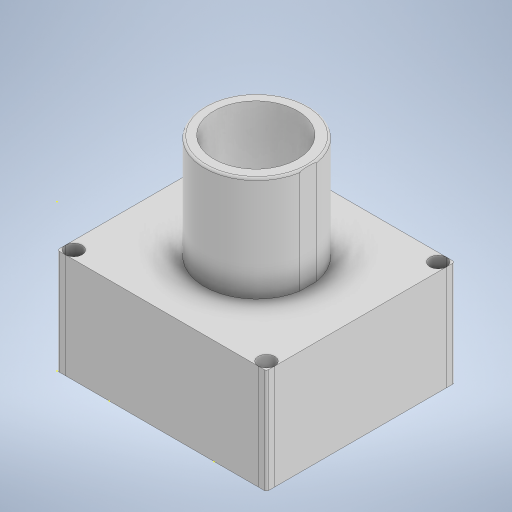
# Autodesk Inventor part: TAREA1_AR
Saved by Autodesk Inventor 2024 (Build 280153000, 153)
## iProperties
Created: 2024-02-15
Part Number: TAREA1_AR
Material: Generic
Document SubType Name: Modeling
Designer: Andreita
Density: 1 g/cm^3
Appearance: Default
Author: Andreita
Autodesk Inventor part; units mm, degrees
ref_plane "YZ Plane" through (0, 0, 0) normal (1, 0, 0) x (0, 1, 0)
ref_plane "XZ Plane" through (0, 0, 0) normal (0, 1, 0) x (-1, 0, 0)
ref_plane "XY Plane" through (0, 0, 0) normal (0, 0, 1) x (1, 0, 0)
sketch "Sketch1" plane through (0, 0, 0) normal (0, 0, 1) x (1, 0, 0)
  line L0 (0, 0) -> (1000, 0)
  line L1 (1000, 0) -> (1000, 500)
  line L2 (1000, 500) -> (0, 500)
  line L3 (0, 500) -> (0, 0)
  line L4 (250, 1000) -> (750, 1000)
  line L5 (250, 1000) -> (250, 500)
  line L6 (750, 1000) -> (750, 500)
  point P0 (80, 250)
  point P1 (0, 250)
  point P2 (1000, 250)
  point P3 (920, 250)
  point P4 (750, 750)
  point P5 (500, 750)
  point P6 (250, 750)
  dimension "d0" = 1000
  dimension "d1" = 500
  dimension "d2" = 80
  dimension "d3" = 80
  dimension "d4" = 1000
  constraints: 14 end point, 4 midpoint, 3 perpendicular, 2 horizontal, 2 parallel, 2 point on line
  measures "d0" distance of L2.end L1.end
  measures "d1" distance of L1.end L0.end
  measures "d2" distance of point (80, 250) point (0, 250)
  measures "d3" distance of point (1000, 250) point (920, 250)
  measures "d4" distance between parallel lines of L1 L3
extrude "Extrusion1" add sketch "Sketch1" against normal blind 900
fillet "Fillet1" radius 10 4 edges at (1000, 250, 0) (0, 250, 0) (0, 250, -900) (1000, 250, -900)
sketch "Sketch2" plane through (0, 0, 0) normal (0, 0, 1) x (1, 0, 0)
  point P0 (0, 0)
sketch "Sketch3" plane through (250, 1000, 0) normal (0, 1, 0) x (1, 0, 0)
  line L0 (500, 0) -> (500, 900) projected
  line L1 (500, 0) -> (0, 0) projected
  circle A0 centre (249.0522, 450) radius 250
  circle A1 centre (249.0522, 450) radius 200
  point P0 (-250, 0)
  point P1 (250, 0)
  constraints: 2 centre point, 2 coincident, 1 midpoint
extrude "Extrusion2" cut sketch "Sketch3" against normal blind 300 contours A1
sketch "Sketch4" plane through (250, 500, 0) normal (-1, 0, 0) x (0, 0, 1)
  point P0 (0, -500)
sketch "Sketch5" plane through (250, 1000, 0) normal (0, 1, 0) x (1, 0, 0)
  circle A0 centre (253.2152, 450) radius 250
  line L0 (500, 0) -> (500, 900) projected
  line L1 (0, 0) -> (500, 0)
  line L2 (500, 0) -> (500, 900)
  line L3 (500, 900) -> (0, 900)
  line L4 (0, 900) -> (0, 0)
  point P0 (-250, 0)
  point P1 (500, 410.0342)
  point P2 (500, 489.9658)
  constraints: 8 end point, 2 parallel, 1 centre point, 1 horizontal, 1 perpendicular
extrude "Extrusion3" cut sketch "Sketch5" against normal blind 500 contours A0 L0 L1 L4 L3
fillet "Fillet2" radius 10 1 edges at (253.2152, 1000, -450)
sketch "Sketch6" plane through (750, 500, -410.0342) normal (1, 0, 0) x (0, 0, -1)
  point P0 (-410.0342, -500)
sketch "Sketch7" plane through (10, 500, 0) normal (0, 1, 0) x (1, 0, 0)
  line L0 (990, 10) -> (990, 890) projected
  line L1 (990, 860) -> (910, 860)
  line L2 (0, 900) -> (980, 900) projected
  line L3 (-10, 10) -> (-10, 890) projected
  line L4 (980, 0) -> (0, 0) projected
  circle A0 centre (30, 860) radius 40
  circle A1 centre (950, 860) radius 40
  circle A2 centre (950, 40) radius 40
  circle A3 centre (30, 40) radius 40
  point P0 (-10, 0)
  point P1 (-10, 450)
  point P2 (30, 455)
  constraints: 3 centre point, 2 end point, 1 horizontal, 1 horizontal alignment, 1 midpoint, 1 point on line, 4 other
extrude "Extrusion4" cut sketch "Sketch7" against normal blind 500 contours A2 | A1 L1 | L1 A1 | A3 | A0
sketch "Sketch8" plane through (499.0522, 700, -450) normal (0, 1, 0) x (1, 0, 0)
  point P0 (-499.0522, -450)
body "Solid1"
